IC202 Holder (Autodesk Fusion 360 design; units mm, degrees)
Autodesk Fusion 360 part; units mm, degrees
note: some values were not read from the file. Chosen so that the rebuilt part matches the saved one: which face or edge a step refers to. Set by a fixed rule: which sketch regions a step uses.
sketch "Sketch1" plane through (0, 0, 0) normal (1, 0, 0) x (0, 1, 0)
  line L0 (-29.5, 25) -> (-29.5, -25)
  line L1 (-29.5, -25) -> (29.5, -25)
  line L2 (29.5, -25) -> (29.5, 25)
  line L3 (29.5, 25) -> (-29.5, -25) construction
  line L4 (-29.5, 25) -> (29.5, -25) construction
  line L5 (-29.5, 25) -> (-36.5577, 25)
  line L6 (-36.5577, 25) -> (-36.5577, -25)
  line L7 (-36.5577, -25) -> (-29.5, -25)
  line L8 (-29.5, -25) -> (-29.5, 25)
  line L9 (36.5577, 25) -> (36.5577, -25)
  line L10 (29.5, 25) -> (36.5577, 25)
  line L11 (36.5577, -25) -> (29.5, -25)
  line L12 (29.5, 25) -> (29.5, -25)
  line L13 (0, -25) -> (-80, -25)
  line L14 (-80, -25) -> (-80, -45)
  line L15 (-80, -45) -> (0, -45)
  line L16 (0, -25) -> (80, -25)
  line L17 (80, -25) -> (80, -45)
  line L18 (80, -45) -> (0, -45)
  line L19 (36.5577, -25) -> (36.5577, -45)
  line L20 (-36.5577, -25) -> (-36.5577, -45)
  line L21 (-80, -40) -> (-36.5577, -40)
  line L22 (36.5577, -40) -> (80, -40)
  dimension "d2" = 50
  dimension "d3" = 7.0577
  dimension "d4" = 80
  dimension "d32" = 80
  dimension "d33" = 5
  dimension "d34" = 5
  constraint parallel L0 L2
  constraint coincident L3 origin
  constraint coincident L4 origin
  constraint horizontal L5
  constraint vertical L6
  constraint horizontal L7
  constraint vertical L8
  constraint horizontal L13
  constraint vertical L14
  constraint horizontal L15
  constraint midpoint L1 L13.start
  constraint coincident L14 L21.start
  constraint coincident L17 L22.end
  constraint perpendicular L17 L21
  constraint coincident L18 L19.end
  constraint perpendicular L18 L19
  constraint coincident L15 L20.end
  constraint perpendicular L15 L20
  constraint coincident L20 L21.end
  constraint coincident L19 L22.start
  constraint collinear L21 L22
  measures "d2" distance of L0.start L0.end
  measures "d3" distance of L0.start L5.end
  measures "d4" distance of L13.start L13.end
  measures "d32" distance of L13.start L17
  measures "d33" distance of L18 L21
  measures "d34" distance of L15 L21
extrude "Extrude1" add sketch "Sketch1" along normal mid plane 60 contours L0 L5 L6 L7 L8 L13 | L2 L9 L10 L11 L12 L16 makes body 1 at (10, 36.5577, 8.3333) makes body 2 at (10, -29.5, 8.3333)
extrude "Extrude2" add sketch "Sketch1" along normal mid plane 100 contours L1 L7 L11 L13 L15 L16 L18 L19 L20 | L13 L14 L20 L21 | L14 L15 L20 L21 | L16 L17 L19 L22 | L17 L18 L19 L22 bodies 1 2
sketch "Sketch2" plane through (0, 36.5577, 0) normal (0, 1, 0) x (-1, 0, 0)
  line L0 (30, 25) -> (-30, 25)
  line L1 (-30, 25) -> (-30, -25)
  line L2 (-30, -25) -> (30, -25)
  line L3 (30, -25) -> (30, 25)
  line L4 (-50, -45) -> (50, -30)
  line L5 (50, -30) -> (50, -45)
  line L6 (50, -45) -> (-50, -45)
  line L7 (50, -30) -> (-50, -30)
  line L8 (-50, -30) -> (-50, -45)
  line L9 (-30, -30) -> (-30, 30)
  circle A0 centre (-30, 30) radius 35
  dimension "d12" = 60
  dimension "d13" = 70
  constraint vertical L5
  constraint perpendicular L5 L6
  constraint perpendicular L5 L7
  constraint perpendicular L7 L8
  constraint coincident L7 L9.start
  constraint perpendicular L2 L9
  constraint coincident L9.end A0.centre
  measures "d12" distance of L9.start L9.end
  measures "d13" diameter of A0
extrude "Extrude3" cut sketch "Sketch2" along normal mid plane 240 contours L4 L5 L6 bodies 1
extrude "Extrude4" cut sketch "Sketch2" against normal blind 15 contours L0 L1 L9 A0 | L0 L1 L9 A0 bodies 1
sketch "Sketch3" plane through (0, 0, 0) normal (0, 0, 1) x (1, 0, 0)
  line L0 (37.0951, -23.8603) -> (-37.0951, -23.8603)
  line L1 (-37.0951, -23.8603) -> (-37.0951, 23.8603)
  line L2 (-37.0951, 23.8603) -> (37.0951, 23.8603)
  line L3 (37.0951, 23.8603) -> (37.0951, -23.8603)
  line L4 (37.0951, -23.8603) -> (-37.0951, 23.8603) construction
  line L5 (-37.0951, -23.8603) -> (37.0951, 23.8603) construction
  line L6 (-70, 0) -> (60, 0)
  line L7 (-37.0951, -42.1663) -> (-37.0951, -73.5722)
  line L8 (37.0951, -42.1663) -> (37.0951, -73.5722)
  line L9 (-37.0951, -73.5722) -> (37.0951, -73.5722)
  line L10 (37.0951, -73.5722) -> (37.0951, -42.1663)
  line L11 (37.0951, -42.1663) -> (-37.0951, -42.1663)
  line L12 (-37.0951, -42.1663) -> (-37.0951, -73.5722)
  line L13 (-37.0951, 42.1663) -> (-37.0951, 73.5722)
  line L14 (37.0951, 42.1663) -> (-37.0951, 42.1663)
  line L15 (37.0951, 73.5722) -> (37.0951, 42.1663)
  line L16 (-37.0951, 73.5722) -> (37.0951, 73.5722)
  constraint horizontal L0
  constraint perpendicular L0 L1
  constraint parallel L0 L2
  constraint parallel L1 L3
  constraint coincident L4 origin
  constraint coincident L5 origin
  constraint horizontal L6
  constraint perpendicular L0 L7
  constraint perpendicular L0 L8
  constraint horizontal L9
  constraint vertical L10
  constraint horizontal L11
  constraint vertical L12
  constraint symmetric L6 L7.end L13.end
  constraint symmetric L6 L8.end L15.start
  constraint symmetric L6 L8.start L14.start
  constraint symmetric L6 L7.start L13.start
extrude "Extrude5" cut sketch "Sketch3" against normal through all contours L0 L1 L3 L6 | L1 L2 L3 L6 bodies 1
fillet "Fillet1" radius 2.5 4 edges at (30, -33.0288, 25) (-30, -33.0288, 25) (-30, 33.0288, 25) (-4.641, 33.0288, 25) on bodies 1 2
fillet "Fillet2" radius 2.5 4 edges at (50, -80, -35) (50, 80, -35) (-50, -80, -27.5) (-50, 80, -27.5) on bodies 1
fillet "Fillet4" radius 2.5 8 edges at (50, 0, -25) (49.2678, -79.2678, -25) (0, -80, -25) (-49.2678, -79.2678, -25) (-50, 0, -25) (-49.2678, 79.2678, -25) (0, 80, -25) (49.2678, 79.2678, -25) on bodies 1
ref_plane "WorkPlane1" through (145, 0, 0) normal (1, 0, 0) x (0, 1, 0)
sketch "Sketch4" plane through (145, 0, 0) normal (1, 0, 0) x (0, 1, 0)
  line L0 (-28.4804, -41.512) -> (-28.4804, -31.512)
  line L1 (-28.4804, -31.512) -> (-27.1571, -31.512)
  line L2 (-27.1571, -31.512) -> (-27.1571, -41.512)
  line L3 (-27.1571, -41.512) -> (-28.4804, -41.512)
  line L4 (-24.8379, -41.512) -> (-24.8379, -31.512)
  line L5 (-24.8379, -31.512) -> (-23.4804, -31.512)
  line L6 (-23.4804, -31.512) -> (-18.228, -39.3633)
  line L7 (-18.228, -39.3633) -> (-18.228, -31.512)
  line L8 (-18.228, -31.512) -> (-16.9593, -31.512)
  line L9 (-16.9593, -31.512) -> (-16.9593, -41.512)
  line L10 (-16.9593, -41.512) -> (-18.3167, -41.512)
  line L11 (-18.3167, -41.512) -> (-23.5691, -33.6539)
  line L12 (-23.5691, -33.6539) -> (-23.5691, -41.512)
  line L13 (-23.5691, -41.512) -> (-24.8379, -41.512)
  line L14 (-15.2267, -38.8722) -> (-13.9988, -38.7085)
  spline S0 degree 3 poles (-13.9988, -38.7085) (-13.9281, -39.02) (-13.8013, -39.5781) (-13.4392, -40.0182) (-13.2792, -40.2126) knots 0 0 0 0 0.094219 0.168777 0.168777 0.168777 0.168777
  spline S1 degree 3 poles (-13.2792, -40.2126) (-13.0985, -40.3469) (-12.7309, -40.6201) (-12.2737, -40.6552) (-12.0411, -40.673) knots 0 0 0 0 0.066099 0.13452 0.13452 0.13452 0.13452
  spline S2 degree 3 poles (-12.0411, -40.673) (-11.7643, -40.6487) (-11.2141, -40.6003) (-10.7891, -40.2478) (-10.578, -40.0727) knots 0 0 0 0 0.081291 0.161533 0.161533 0.161533 0.161533
  spline S3 degree 3 poles (-10.578, -40.0727) (-10.4039, -39.8588) (-10.0511, -39.4254) (-10.0047, -38.868) (-9.9811, -38.5857) knots 0 0 0 0 0.080736 0.163605 0.163605 0.163605 0.163605
  spline S4 degree 3 poles (-9.9811, -38.5857) (-10.0019, -38.3183) (-10.0426, -37.7957) (-10.3725, -37.3893) (-10.5336, -37.1907) knots 0 0 0 0 0.078392 0.15324 0.15324 0.15324 0.15324
  spline S5 degree 3 poles (-10.5336, -37.1907) (-10.7338, -37.0306) (-11.1444, -36.702) (-11.6696, -36.6621) (-11.9388, -36.6416) knots 0 0 0 0 0.075063 0.154028 0.154028 0.154028 0.154028
  spline S6 degree 3 poles (-11.9388, -36.6416) (-12.0695, -36.6494) (-12.3625, -36.6668) (-12.6474, -36.7384) (-12.8051, -36.7781) knots 0 0 0 0 0.0392 0.087867 0.087867 0.087867 0.087867
  line L15 (-12.8051, -36.7781) -> (-12.6687, -35.7003)
  spline S7 degree 3 poles (-12.6687, -35.7003) (-12.6318, -35.7043) (-12.566, -35.7113) (-12.4999, -35.7131) (-12.4709, -35.7139) knots 0 0 0 0 0.011132 0.019836 0.019836 0.019836 0.019836
  spline S8 degree 3 poles (-12.4709, -35.7139) (-12.2172, -35.6977) (-11.7161, -35.6657) (-11.2762, -35.424) (-11.0589, -35.3047) knots 0 0 0 0 0.075222 0.148626 0.148626 0.148626 0.148626
  spline S9 degree 3 poles (-11.0589, -35.3047) (-10.8759, -35.1446) (-10.4952, -34.8115) (-10.4532, -34.3055) (-10.4313, -34.0427) knots 0 0 0 0 0.070147 0.145969 0.145969 0.145969 0.145969
  spline S10 degree 3 poles (-10.4313, -34.0427) (-10.4491, -33.8286) (-10.484, -33.4072) (-10.7551, -33.0833) (-10.8883, -32.924) knots 0 0 0 0 0.062781 0.123515 0.123515 0.123515 0.123515
  spline S11 degree 3 poles (-10.8883, -32.924) (-11.0558, -32.7948) (-11.403, -32.5267) (-11.8414, -32.4964) (-12.0684, -32.4807) knots 0 0 0 0 0.062022 0.128606 0.128606 0.128606 0.128606
  spline S12 degree 3 poles (-12.0684, -32.4807) (-12.2952, -32.4975) (-12.7379, -32.5304) (-13.0903, -32.7996) (-13.2622, -32.9309) knots 0 0 0 0 0.066612 0.130061 0.130061 0.130061 0.130061
  spline S13 degree 3 poles (-13.2622, -32.9309) (-13.4086, -33.111) (-13.7297, -33.5062) (-13.8245, -34.0083) (-13.8761, -34.2815) knots 0 0 0 0 0.068596 0.150441 0.150441 0.150441 0.150441
  line L16 (-13.8761, -34.2815) -> (-15.1039, -34.0632)
  spline S14 degree 3 poles (-15.1039, -34.0632) (-15.0121, -33.6811) (-14.8371, -32.9526) (-14.3244, -32.4085) (-14.0807, -32.1498) knots 0 0 0 0 0.115593 0.220352 0.220352 0.220352 0.220352
  spline S15 degree 3 poles (-14.0807, -32.1498) (-13.7921, -31.9519) (-13.1945, -31.5421) (-12.4702, -31.4953) (-12.0957, -31.4711) knots 0 0 0 0 0.102989 0.213272 0.213272 0.213272 0.213272
  spline S16 degree 3 poles (-12.0957, -31.4711) (-11.83, -31.4849) (-11.3064, -31.512) (-10.8252, -31.7199) (-10.5882, -31.8224) knots 0 0 0 0 0.079104 0.1559 0.1559 0.1559 0.1559
  spline S17 degree 3 poles (-10.5882, -31.8224) (-10.3736, -31.9477) (-9.954, -32.1926) (-9.672, -32.5878) (-9.5343, -32.7808) knots 0 0 0 0 0.073622 0.143898 0.143898 0.143898 0.143898
  spline S18 degree 3 poles (-9.5343, -32.7808) (-9.4279, -32.9851) (-9.2171, -33.3898) (-9.1852, -33.8448) (-9.1694, -34.07) knots 0 0 0 0 0.068309 0.13527 0.13527 0.13527 0.13527
  spline S19 degree 3 poles (-9.1694, -34.07) (-9.1836, -34.2807) (-9.2118, -34.7) (-9.4158, -35.0674) (-9.5173, -35.2501) knots 0 0 0 0 0.062511 0.124386 0.124386 0.124386 0.124386
  spline S20 degree 3 poles (-9.5173, -35.2501) (-9.6518, -35.4204) (-9.9332, -35.7768) (-10.3367, -35.9865) (-10.5473, -36.0959) knots 0 0 0 0 0.064354 0.134636 0.134636 0.134636 0.134636
  spline S21 degree 3 poles (-10.5473, -36.0959) (-10.271, -36.1789) (-9.7353, -36.3397) (-9.354, -36.7477) (-9.1694, -36.9452) knots 0 0 0 0 0.084836 0.164458 0.164458 0.164458 0.164458
  spline S22 degree 3 poles (-9.1694, -36.9452) (-9.0262, -37.1807) (-8.7254, -37.6755) (-8.6945, -38.2548) (-8.6783, -38.5584) knots 0 0 0 0 0.081375 0.170983 0.170983 0.170983 0.170983
  spline S23 degree 3 poles (-8.6783, -38.5584) (-8.7184, -38.9787) (-8.7988, -39.821) (-9.3547, -40.459) (-9.6332, -40.7787) knots 0 0 0 0 0.123326 0.247176 0.247176 0.247176 0.247176
  spline S24 degree 3 poles (-9.6332, -40.7787) (-9.9791, -41.0443) (-10.6908, -41.5908) (-11.5872, -41.6559) (-12.048, -41.6894) knots 0 0 0 0 0.127883 0.263168 0.263168 0.263168 0.263168
  spline S25 degree 3 poles (-12.048, -41.6894) (-12.4631, -41.6611) (-13.2675, -41.6064) (-13.919, -41.1337) (-14.2342, -40.9049) knots 0 0 0 0 0.122066 0.236491 0.236491 0.236491 0.236491
  spline S26 degree 3 poles (-14.2342, -40.9049) (-14.4933, -40.6203) (-15.0216, -40.04) (-15.1575, -39.2664) (-15.2267, -38.8722) knots 0 0 0 0 0.113013 0.230401 0.230401 0.230401 0.230401
  line L17 (-8.0643, -41.512) -> (-4.224, -31.512)
  line L18 (-4.224, -31.512) -> (-2.7983, -31.512)
  line L19 (-2.7983, -31.512) -> (1.2945, -41.512)
  line L20 (1.2945, -41.512) -> (-0.213, -41.512)
  line L21 (-0.213, -41.512) -> (-1.3795, -38.4834)
  line L22 (-1.3795, -38.4834) -> (-5.5609, -38.4834)
  line L23 (-5.5609, -38.4834) -> (-6.6591, -41.512)
  line L24 (-6.6591, -41.512) -> (-8.0643, -41.512)
  line L25 (-5.1789, -37.4056) -> (-1.7888, -37.4056)
  line L26 (-1.7888, -37.4056) -> (-2.8324, -34.6362)
  spline S27 degree 3 poles (-2.8324, -34.6362) (-2.9754, -34.2545) (-3.2319, -33.5701) (-3.4468, -32.8715) (-3.5418, -32.5625) knots 0 0 0 0 0.122238 0.219209 0.219209 0.219209 0.219209
  spline S28 degree 3 poles (-3.5418, -32.5625) (-3.6124, -32.8837) (-3.7548, -33.5309) (-3.9715, -34.1571) (-4.0807, -34.4725) knots 0 0 0 0 0.098565 0.198603 0.198603 0.198603 0.198603
  line L27 (-4.0807, -34.4725) -> (-5.1789, -37.4056)
  spline S29 degree 3 poles (9.9302, -40.4411) (10.2199, -40.6339) (10.7592, -40.9929) (11.3536, -41.2499) (11.6287, -41.3688) knots 0 0 0 0 0.104157 0.193879 0.193879 0.193879 0.193879
  line L28 (11.6287, -41.3688) -> (11.2399, -42.2897)
  spline S30 degree 3 poles (11.2399, -42.2897) (10.8738, -42.1356) (10.1081, -41.8135) (9.4399, -41.3196) (9.0912, -41.0618) knots 0 0 0 0 0.118712 0.248263 0.248263 0.248263 0.248263
  spline S31 degree 3 poles (9.0912, -41.0618) (8.7078, -41.2429) (7.9301, -41.6101) (7.0711, -41.6582) (6.6355, -41.6826) knots 0 0 0 0 0.125908 0.255422 0.255422 0.255422 0.255422
  spline S32 degree 3 poles (6.6355, -41.6826) (6.1963, -41.6569) (5.3306, -41.6063) (4.5551, -41.2187) (4.173, -41.0277) knots 0 0 0 0 0.130465 0.257184 0.257184 0.257184 0.257184
  spline S33 degree 3 poles (4.173, -41.0277) (3.825, -40.7855) (3.1226, -40.2968) (2.6896, -39.5584) (2.4711, -39.186) knots 0 0 0 0 0.125587 0.253443 0.253443 0.253443 0.253443
  spline S34 degree 3 poles (2.4711, -39.186) (2.2971, -38.771) (1.9385, -37.9159) (1.8961, -36.989) (1.8743, -36.512) knots 0 0 0 0 0.133898 0.275885 0.275885 0.275885 0.275885
  spline S35 degree 3 poles (1.8743, -36.512) (1.8969, -36.0346) (1.9411, -35.1013) (2.2995, -34.2389) (2.4745, -33.8176) knots 0 0 0 0 0.142165 0.277918 0.277918 0.277918 0.277918
  spline S36 degree 3 poles (2.4745, -33.8176) (2.6928, -33.4388) (3.1227, -32.6928) (3.8335, -32.2078) (4.1833, -31.9691) knots 0 0 0 0 0.129316 0.254636 0.254636 0.254636 0.254636
  spline S37 degree 3 poles (4.1833, -31.9691) (4.5678, -31.784) (5.3515, -31.407) (6.2203, -31.3591) (6.6628, -31.3347) knots 0 0 0 0 0.126685 0.258187 0.258187 0.258187 0.258187
  spline S38 degree 3 poles (6.6628, -31.3347) (7.1095, -31.36) (7.9869, -31.4099) (8.7733, -31.801) (9.1594, -31.9929) knots 0 0 0 0 0.132675 0.260594 0.260594 0.260594 0.260594
  spline S39 degree 3 poles (9.1594, -31.9929) (9.5085, -32.2353) (10.2107, -32.7228) (10.6391, -33.4627) (10.8545, -33.8347) knots 0 0 0 0 0.125827 0.253061 0.253061 0.253061 0.253061
  spline S40 degree 3 poles (10.8545, -33.8347) (11.0246, -34.2491) (11.3756, -35.1045) (11.4166, -36.0287) (11.4377, -36.5052) knots 0 0 0 0 0.133318 0.275184 0.275184 0.275184 0.275184
  spline S41 degree 3 poles (11.4377, -36.5052) (11.4248, -36.8992) (11.3999, -37.6566) (11.1719, -38.3789) (11.0625, -38.7255) knots 0 0 0 0 0.117615 0.226119 0.226119 0.226119 0.226119
  spline S42 degree 3 poles (11.0625, -38.7255) (10.9217, -39.0433) (10.6401, -39.6785) (10.1667, -40.187) (9.9302, -40.4411) knots 0 0 0 0 0.103494 0.206836 0.206836 0.206836 0.206836
  spline S43 degree 3 poles (7.0175, -38.7494) (7.3757, -38.8635) (8.0574, -39.0806) (8.6336, -39.5036) (8.907, -39.7044) knots 0 0 0 0 0.111893 0.212969 0.212969 0.212969 0.212969
  spline S44 degree 3 poles (8.907, -39.7044) (9.2466, -39.2789) (9.9889, -38.3488) (10.0437, -37.1537) (10.0735, -36.5052) knots 0 0 0 0 0.159348 0.348343 0.348343 0.348343 0.348343
  spline S45 degree 3 poles (10.0735, -36.5052) (10.06, -36.1219) (10.0345, -35.3923) (9.7811, -34.7084) (9.6608, -34.3838) knots 0 0 0 0 0.114212 0.217362 0.217362 0.217362 0.217362
  spline S46 degree 3 poles (9.6608, -34.3838) (9.5094, -34.0997) (9.2114, -33.5402) (8.7034, -33.1615) (8.4534, -32.9752) knots 0 0 0 0 0.095263 0.187581 0.187581 0.187581 0.187581
  spline S47 degree 3 poles (8.4534, -32.9752) (8.1782, -32.829) (7.6203, -32.5325) (6.9894, -32.4936) (6.6696, -32.4738) knots 0 0 0 0 0.092332 0.187212 0.187212 0.187212 0.187212
  spline S48 degree 3 poles (6.6696, -32.4738) (6.1997, -32.5135) (5.2732, -32.5918) (4.5636, -33.1914) (4.214, -33.4868) knots 0 0 0 0 0.13775 0.27157 0.27157 0.27157 0.27157
  spline S49 degree 3 poles (4.214, -33.4868) (3.9302, -33.894) (3.3004, -34.7976) (3.2605, -35.9041) (3.2385, -36.512) knots 0 0 0 0 0.14594 0.323864 0.323864 0.323864 0.323864
  spline S50 degree 3 poles (3.2385, -36.512) (3.2628, -37.1059) (3.3073, -38.1985) (3.9228, -39.0966) (4.2037, -39.5066) knots 0 0 0 0 0.174088 0.320312 0.320312 0.320312 0.320312
  spline S51 degree 3 poles (4.2037, -39.5066) (4.5515, -39.811) (5.258, -40.4292) (6.1943, -40.5095) (6.6696, -40.5502) knots 0 0 0 0 0.134932 0.274081 0.274081 0.274081 0.274081
  spline S52 degree 3 poles (6.6696, -40.5502) (6.9016, -40.5396) (7.3608, -40.5186) (7.7928, -40.3618) (8.0066, -40.2842) knots 0 0 0 0 0.069215 0.13702 0.13702 0.13702 0.13702
  spline S53 degree 3 poles (8.0066, -40.2842) (7.7981, -40.16) (7.3854, -39.9143) (6.9248, -39.7784) (6.6969, -39.7112) knots 0 0 0 0 0.072487 0.143456 0.143456 0.143456 0.143456
  line L29 (6.6969, -39.7112) -> (7.0175, -38.7494)
  line L30 (13.1635, -41.512) -> (13.1635, -31.512)
  line L31 (13.1635, -31.512) -> (14.4868, -31.512)
  line L32 (14.4868, -31.512) -> (14.4868, -36.4711)
  line L33 (14.4868, -36.4711) -> (19.4527, -31.512)
  line L34 (19.4527, -31.512) -> (21.2467, -31.512)
  line L35 (21.2467, -31.512) -> (17.0516, -35.5639)
  line L36 (17.0516, -35.5639) -> (21.4309, -41.512)
  line L37 (21.4309, -41.512) -> (19.6846, -41.512)
  line L38 (19.6846, -41.512) -> (16.1239, -36.4506)
  line L39 (16.1239, -36.4506) -> (14.4868, -38.0468)
  line L40 (14.4868, -38.0468) -> (14.4868, -41.512)
  line L41 (14.4868, -41.512) -> (13.1635, -41.512)
fillet "Fillet6" radius 10 4 edges at (37.0951, 23.8603, -34.0321) (37.0951, -23.8603, -34.0321) (-37.0951, -23.8603, -28.4679) (-37.0951, 23.8603, -28.4679) on bodies 1
extrude "Extrude10" cut sketch "Sketch3" against normal through all contours L7 L8 L9 L10 L11 L12 | L13 L14 L15 L16 bodies 1
fillet "Fillet7" radius 10 4 edges at (-37.0951, -73.5722, -28.4679) (-37.0951, -42.1663, -28.4679) (37.0951, -73.5722, -34.0321) (37.0951, -42.1663, -34.0321) on bodies 1
fillet "Fillet8" radius 10 4 edges at (-37.0951, 42.1663, -28.4679) (37.0951, 42.1663, -34.0321) (37.0951, 73.5722, -34.0321) (-37.0951, 73.5722, -28.4679) on bodies 1
extrude "Extrude11" cut sketch "Sketch4" against normal blind 99 bodies 1
chamfer "Chamfer4" distance 5 angle 45 2 edges at (0, 36.5577, -25) (0, -36.5577, -25) on bodies 1
